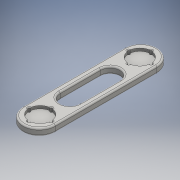
# Autodesk Inventor part: LowerArm
Saved by Autodesk Inventor 2016 (Build 200138000, 138)
## iProperties
Created: 2015-10-06
Part Number: LowerArm
Material: Generic
Document SubType Name: Modeling
Designer: alex
Density: 1 g/cm^3
Appearance: Default
Mass: 56.6565 g
Surface Area: 198.211 cm^2
Volume: 56.6565 cm^3
Author: alex
Autodesk Inventor part; units mm, degrees
ref_plane "YZ Plane" through (0, 0, 0) normal (1, 0, 0) x (0, 1, 0)
ref_plane "XZ Plane" through (0, 0, 0) normal (0, 1, 0) x (-1, 0, 0)
ref_plane "XY Plane" through (0, 0, 0) normal (0, 0, 1) x (1, 0, 0)
sketch "Sketch1" plane through (0, 0, 0) normal (0, 0, 1) x (1, 0, 0)
  line L0 (-20, 83) -> (20, 83)
  line L1 (20, 83) -> (20, -83)
  line L2 (20, -83) -> (-20, -83)
  line L3 (-20, -83) -> (-20, 83)
  point P0 (0, 0)
  dimension "d0" = 83
  dimension "d1" = 83
  dimension "d2" = 20
  dimension "d3" = 20
  constraints: 8 end point, 2 parallel, 1 horizontal, 1 perpendicular
  measures "d0" distance from line of point (0, 0) L0
  measures "d1" distance from line of point (0, 0) L2
  measures "d2" distance from line of point (0, 0) L3
  measures "d3" distance from line of point (0, 0) L1
extrude "Extrusion1" add sketch "Sketch1" along normal blind 9
fillet "Fillet1" radius 20 1 edges at (-20, 83, 4.5)
fillet "Fillet2" radius 20 1 edges at (20, 83, 4.5)
mirror "Mirror1" about plane through (0, 0, 0) normal (0, 1, 0) of "Fillet1", "Fillet2"
fillet "Fillet6" radius 2 8 edges at (14.1422, 77.1422, 0) (-14.1421, 77.1421, 0) (0, 83, 0) (-20, 0, 0) (0.0001, -83, 0) (14.1422, -77.1422, 0) (-14.1421, -77.1421, 0) (20, 0, 0)
fillet "Fillet7" radius 2 8 edges at (14.1422, 77.1422, 9) (0, 83, 9) (-14.1421, 77.1421, 9) (20, 0, 9) (14.1422, -77.1422, 9) (0.0001, -83, 9) (-14.1421, -77.1421, 9) (-20, 0, 9)
sketch "Sketch6" plane through (0, 0, 9) normal (0, 0, 1) x (1, 0, 0)
  circle A0 centre (0, -61.75) radius 13.75
  arc A1 (-18, -63) -> (18, -63) centre (0, -63) ccw projected
  line L0 (18, 63) -> (18, -63) projected
  circle A2 centre (0, -48) radius 1.5
  circle A3 centre (-13.75, -61.75) radius 1.5
  circle A4 centre (0, -75.5) radius 1.5
  circle A5 centre (13.75, -61.75) radius 1.5
  line L1 (0, 0) -> (-53.5469, 0)
  circle A6 centre (0, 61.75) radius 13.75
  circle A7 centre (0, 48) radius 1.5
  circle A8 centre (-13.75, 61.75) radius 1.5
  circle A9 centre (0, 75.5) radius 1.5
  circle A10 centre (13.75, 61.75) radius 1.5
  dimension "d41" = 27.5
  dimension "d42" = 5.5
  dimension "d43" = 18
  dimension "d44" = 3
  dimension "d45" = 13.75
  dimension "d46" = 18
  dimension "d49" = 360
  constraints: 10 centre point, 5 symmetric about line, 2 end point, 1 horizontal, 14 other
  measures "d41" diameter of A0
  measures "d43" distance from line of L0 A0.centre
  measures "d44" diameter of A2
  measures "d45" distance of A0.centre A2.centre
  measures "d46" distance from line of L0 A2.centre
extrude "Extrusion6" cut sketch "Sketch6" against normal through all contours A0 A5 | A0 A5 | A2 A0 | A0 A2 | A4 A0 | A0 A4 | A3 A0 | A0 A3 | A6 A10 | A6 A10 | A9 A6 | A6 A9 | A7 A6 | A6 A7 | A8 A6 | A6 A8
fillet "Fillet8" radius 1 16 edges at (-15.25, 61.75, 9) (-1.5, 75.5, 9) (12.25, 61.75, 9) (-1.5, 48, 9) (-1.5, -75.5, 9) (-15.25, -61.75, 9) (-1.5, -48, 9) (12.25, -61.75, 9) (12.25, -61.75, 0) (-1.5, -75.5, 0) (-1.5, -48, 0) (-15.25, -61.75, 0) (12.25, 61.75, 0) (-1.5, 48, 0) (-15.25, 61.75, 0) (-1.5, 75.5, 0)
sketch "Sketch8" plane through (0, 0, 9) normal (0, 0, 1) x (1, 0, 0)
  circle A0 centre (0, -61.75) radius 13.75
  line L0 (-18, -63) -> (-18, 63) projected
  arc A1 (-18, -63) -> (18, -63) centre (0, -63) ccw projected
  line L1 (0, 0) -> (-37.1861, 0)
  circle A2 centre (0, 61.75) radius 13.75
  dimension "d62" = 27.5
  dimension "d63" = 18
  dimension "d64" = 1.25
  constraints: 2 centre point, 2 end point, 1 horizontal, 1 symmetric about line, 1 other
  measures "d62" diameter of A0
  measures "d63" distance from line of L0 A0.centre
  measures "d64" distance of A1.centre A0.centre
extrude "Extrusion8" cut sketch "Sketch8" against normal blind 3.5
sketch "Sketch9" plane through (0, 0, 9) normal (0, 0, 1) x (1, 0, 0)
  line L0 (12, -25.0296) -> (12, 24.9704)
  line L1 (-12, 24.9704) -> (-12, -25.0296)
  line L2 (-18, 63) -> (-18, -63) projected
  line L3 (18, 63) -> (18, -63) projected
  arc A0 (12, 24.9704) -> (-12, 24.9704) centre (0, 24.9704) ccw
  arc A1 (-12, -25.0296) -> (12, -25.0296) centre (0, -25.0296) ccw
  point P0 (0, 0)
  dimension "d67" = 6
  dimension "d68" = 6
  dimension "d71" = 24
  dimension "d72" = 24
  dimension "d73" = 50
  dimension "d74" = 38.5
  constraints: 4 end point, 4 point on circle, 2 centre point, 2 tangent, 1 parallel
  measures "d67" distance between parallel lines of L2 L1
  measures "d68" distance between parallel lines of L3 L0
  measures "d71" diameter of A0
  measures "d72" diameter of A1
  measures "d73" distance of A0.centre A1.centre
  measures "d74" distance of L3.start L0.end
extrude "Extrusion9" cut sketch "Sketch9" against normal through all
fillet "Fillet10" radius 2 8 edges at (0, 36.9704, 9) (12, -0.0296, 9) (0, -37.0296, 9) (-12, -0.0296, 9) (0, -37.0296, 0) (12, -0.0296, 0) (0, 36.9704, 0) (-12, -0.0296, 0)
body "Solid1"
